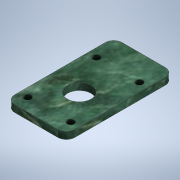
# Autodesk Inventor part: potentiometerpcb
Saved by Autodesk Inventor 2020 (Build 240168000, 168)
## iProperties
Created: 2020-01-19
Part Number: potentiometerpcb
Material: Generic
Document SubType Name: Modeling
Designer: sami_
Density: 1 g/cm^3
Appearance: Green Polished
Author: sami_
Autodesk Inventor part; units mm, degrees
ref_plane "YZ Plane" through (0, 0, 0) normal (1, 0, 0) x (0, 1, 0)
ref_plane "XZ Plane" through (0, 0, 0) normal (0, 1, 0) x (-1, 0, 0)
ref_plane "XY Plane" through (0, 0, 0) normal (0, 0, 1) x (1, 0, 0)
sketch "Sketch1" plane through (0, 0, 0) normal (0, 1, 0) x (-1, 0, 0)
  line L0 (-4.5005, -6.5) -> (-3.283, -6.5)
  line L1 (-3.283, -6.5) -> (-2.9693, -6.948)
  line L2 (-2.9693, -6.948) -> (-2.9693, -8.2299)
  line L3 (-2.9693, -8.2299) -> (-2.0718, -8.2299)
  line L4 (-2.0718, -8.2299) -> (-2.0718, -7.0351)
  line L5 (-2.0718, -7.0351) -> (-1.8086, -6.5)
  line L6 (-1.8086, -6.5) -> (-0.6909, -6.5)
  line L7 (-0.6909, -6.5) -> (-0.4278, -7.0351)
  line L8 (-0.4278, -7.0351) -> (-0.4278, -8.2299)
  line L9 (-0.4278, -8.2299) -> (0.4698, -8.2299)
  line L10 (0.4698, -8.2299) -> (0.4698, -6.948)
  line L11 (0.4698, -6.948) -> (0.7835, -6.5)
  line L12 (0.7835, -6.5) -> (1.8077, -6.5)
  line L13 (1.8077, -6.5) -> (2.0708, -7.0351)
  line L14 (2.0708, -7.0351) -> (2.0708, -8.2299)
  line L15 (2.0708, -8.2299) -> (2.9683, -8.2299)
  line L16 (2.9683, -8.2299) -> (2.9683, -6.948)
  line L17 (2.9683, -6.948) -> (3.2821, -6.5)
  line L18 (3.2821, -6.5) -> (4.4995, -6.5)
  line L19 (4.4995, -6.5) -> (5.4995, -5.5)
  line L20 (5.4995, -5.5) -> (5.4995, 1.9247)
  line L21 (5.4995, 1.9247) -> (2.4995, 5.5)
  line L22 (2.4995, 5.5) -> (0.4698, 5.5)
  line L23 (0.4698, 5.5) -> (0.4698, 6.6191)
  line L24 (0.4698, 6.6191) -> (-0.4278, 6.6191)
  line L25 (-0.4278, 6.6191) -> (-0.4278, 5.5)
  line L26 (-0.4278, 5.5) -> (-2.5005, 5.5)
  line L27 (-2.5005, 5.5) -> (-5.5005, 1.9247)
  line L28 (-5.5005, 1.9247) -> (-5.5005, -5.5)
  line L29 (-5.5005, -5.5) -> (-4.5005, -6.5)
  circle A0 centre (-0.0005, -2.3274) radius 0.7145
  line L30 (6.998, 7.6726) -> (-7.002, 7.6726)
  line L31 (-7.002, 7.6726) -> (-7.002, -17.3274)
  line L32 (-7.002, -17.3274) -> (6.998, -17.3274)
  line L33 (6.998, -17.3274) -> (6.998, 7.6726)
  circle A1 centre (-0.0005, -2.3274) radius 2.75
  line L34 (-0.002, -21.2436) -> (-0.002, 13.4129) construction
  point P0 (-0.002, -0.846)
  dimension "d0" = 14
  dimension "d1" = 25
  dimension "d2" = 5.5
  dimension "d19" = 7
  dimension "d22" = 10
  constraints: 70 end point, 2 centre point, 2 parallel, 1 coincident, 1 horizontal, 1 perpendicular, 1 point on line, 1 vertical
  measures "d0" distance of L32.end L31.end
  measures "d1" distance of L31.end L30.end
  measures "d2" diameter of A1
  measures "d19" distance between parallel lines of L34 L33
  measures "d22" distance from line of L30 A0.centre
extrude "Extrusion1" add sketch "Sketch1" along normal blind 1.6 contours L29 L28 L27 L26 L25 L24 L23 L22 L21 L20 L19 L18 L17 L16 L15 L14 L13 L12 L11 L10 L9 L8 L7 L6 L5 L4 L3 L2 L1 L0 | L33 L32 L31 L30
sketch "Sketch2" plane through (0, 1.6, 0) normal (0, 1, 0) x (1, 0, 0)
  line L0 (-6.998, 17.3274) -> (-6.998, -7.6726) projected
  line L1 (7.002, 17.3274) -> (-6.998, 17.3274) projected
  line L2 (-6.998, -7.6726) -> (7.002, -7.6726)
  line L3 (7.002, -7.6726) -> (7.002, 17.3274)
  line L4 (7.002, 17.3274) -> (-6.998, 17.3274)
  line L5 (-6.998, 17.3274) -> (-6.998, -7.6726)
  circle A0 centre (5.002, -4.6726) radius 0.8
  circle A1 centre (5.002, 11.3274) radius 0.8
  circle A2 centre (-4.998, 11.3274) radius 0.8
  circle A3 centre (-4.998, -4.6726) radius 0.8
  point P0 (0, 0)
  dimension "d5" = 1.6
  dimension "d6" = 1.6
  dimension "d7" = 1.6
  dimension "d8" = 1.6
  dimension "d9" = 2
  dimension "d10" = 3
  dimension "d11" = 3
  dimension "d12" = 2
  dimension "d13" = 2
  dimension "d15" = 2
  dimension "d20" = 16
  dimension "d21" = 16
  constraints: 8 end point, 4 centre point, 2 parallel, 1 horizontal, 1 perpendicular
  measures "d5" diameter of A0
  measures "d6" diameter of A1
  measures "d7" diameter of A2
  measures "d8" diameter of A3
  measures "d9" distance from line of L3 A0.centre
  measures "d10" distance from line of L2 A0.centre
  measures "d11" distance from line of L2 A3.centre
  measures "d12" distance from line of L0 A3.centre
  measures "d13" distance from line of L5 A2.centre
  measures "d15" distance from line of L3 A1.centre
  measures "d20" distance of A0.centre A1.centre
  measures "d21" distance of A3.centre A2.centre
extrude "Extrusion2" cut sketch "Sketch2" against normal blind 1.6 contours A0 | A1 | A2 | A3
fillet "Fillet1" radius 2 4 edges at (-6.998, 0.8, 7.6726) (7.002, 0.8, 7.6726) (-6.998, 0.8, -17.3274) (7.002, 0.8, -17.3274)
equation "\"d19\" = 0.5 * d0"
equation "\"d5\" = d7"
equation "\"d6\" = d7"
equation "\"d8\" = d7"
equation "\"d10\" = d11"
equation "\"d20\" = d21"
body "Solid1"
